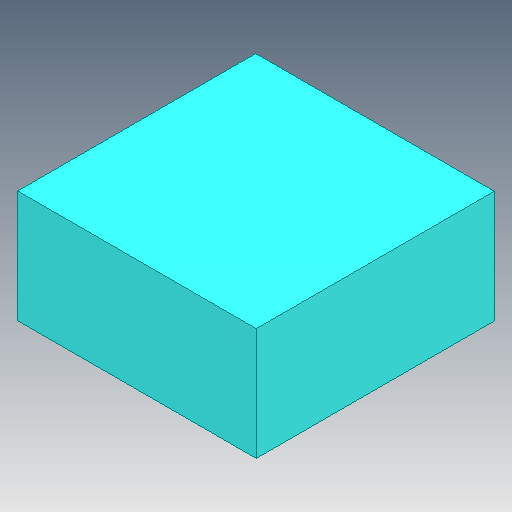
# Autodesk Inventor part: SOLDERJUMPERNC3
Saved by Autodesk Inventor 2017 (Build 210142000, 142)
## iProperties
Part Number: SOLDERJUMPERNC3
Material: Generisch
Document SubType Name: Modeling
Designer: Werkstatt
Density: 1 g/cm^3
Appearance: SJ_2S-NOTRACE, SOLDERJUMPERNC3
Author: Werkstatt
Autodesk Inventor part; units mm, degrees
ref_plane "YZ Plane" through (0, 0, 0) normal (1, 0, 0) x (0, 1, 0)
ref_plane "XZ Plane" through (0, 0, 0) normal (0, 1, 0) x (-1, 0, 0)
ref_plane "XY Plane" through (0, 0, 0) normal (0, 0, 1) x (1, 0, 0)
sketch "SJ_2S-NOTRACE, SOLDERJUMPERNC3_53" plane through (0, 0, 0) normal (0, 0, 1) x (1, 0, 0)
  line L0 (-1.1066, 1.016) -> (1.016, 1.016)
  line L1 (1.016, 1.016) -> (1.016, -1.1016)
  line L2 (1.016, -1.1016) -> (-1.1066, -1.1016)
  line L3 (-1.1066, -1.1016) -> (-1.1066, 1.016)
  constraints: 8 end point
extrude "Extrusion1" add sketch "SJ_2S-NOTRACE, SOLDERJUMPERNC3_53" along normal blind 1
